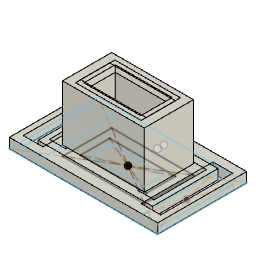
DrVape_DrStick v1 (Autodesk Fusion 360 design; units mm, degrees)
Autodesk Fusion 360 part; units mm, degrees
sketch "スケッチ1" plane through (0, 0, 0) normal (0, 0, 1) x (1, 0, 0)
  line L0 (7.7, 3.8) -> (-7.7, 3.8)
  line L1 (-7.7, 3.8) -> (-7.7, -3.8)
  line L2 (-7.7, -3.8) -> (7.7, -3.8)
  line L3 (7.7, -3.8) -> (7.7, 3.8)
  line L4 (7.7, 3.8) -> (-7.7, -3.8) construction
  line L5 (-7.7, 3.8) -> (7.7, -3.8) construction
  line L6 (10, -6) -> (-10, -6)
  line L7 (-10, -6) -> (-10, 6)
  line L8 (-10, 6) -> (10, 6)
  line L9 (10, 6) -> (10, -6)
  line L10 (10, -6) -> (-10, 6) construction
  line L11 (-10, -6) -> (10, 6) construction
  line L12 (17.5, -10) -> (-17.5, -10)
  line L13 (-17.5, -10) -> (-17.5, 10)
  line L14 (-17.5, 10) -> (17.5, 10)
  line L15 (17.5, 10) -> (17.5, -10)
  line L16 (17.5, -10) -> (-17.5, 10) construction
  line L17 (-17.5, -10) -> (17.5, 10) construction
  dimension "d1" = 15.4
  dimension "d2" = 7.6
  dimension "d3" = 20
  dimension "d4" = 12
  dimension "d5" = 35
  dimension "d6" = 20
  constraint horizontal L0
  constraint perpendicular L0 L1
  constraint parallel L0 L2
  constraint parallel L1 L3
  constraint coincident L4 origin
  constraint coincident L5 origin
  constraint horizontal L6
  constraint perpendicular L6 L7
  constraint parallel L6 L8
  constraint parallel L7 L9
  constraint coincident L10 origin
  constraint coincident L11 origin
  constraint horizontal L12
  constraint perpendicular L12 L13
  constraint parallel L12 L14
  constraint parallel L13 L15
  constraint coincident L16 origin
  constraint coincident L17 origin
  measures "d1" distance of L1.end L2.end
  measures "d2" distance of L0.end L1.end
  measures "d3" distance of L7.end L8.end
  measures "d4" distance of L6.end L7.end
  measures "d5" distance of L13.end L14.end
  measures "d6" distance of L12.end L13.end
extrude "押し出し1" add sketch "スケッチ1" along normal blind 20 contours L6 L7 L8 L9 makes body 1
extrude "押し出し2" add sketch "スケッチ1" along normal blind 3 contours L0 L1 L2 L3 | L6 L7 L8 L9 | L12 L13 L14 L15 bodies 1
chamfer "面取り1" distance 1 angle 45 4 edges at (0, 3.8, 20) (-7.7, 0, 20) (0, -3.8, 20) (7.7, 0, 20) on bodies 1
sketch "スケッチ2" plane through (0, 0, 3) normal (0, 0, 1) x (-1, 0, 0)
  line L0 (-17.5, -10) -> (17.5, -10)
  line L1 (17.5, -10) -> (17.5, 10)
  line L2 (17.5, 10) -> (-17.5, 10)
  line L3 (-17.5, 10) -> (-17.5, -10)
  line L4 (-10, -6) -> (-10, 6)
  line L5 (-10, 6) -> (10, 6)
  line L6 (10, 6) -> (10, -6)
  line L7 (10, -6) -> (-10, -6)
  line L8 (-11, -8) -> (-16, -8)
  line L9 (-16, -8) -> (-16, 8)
  line L10 (-16, 8) -> (-11, 8)
  line L11 (-11, 8) -> (-11, -8)
  line L12 (0, -7) -> (0, -1)
  line L13 (11, 8) -> (11, -8)
  line L14 (11, -8) -> (16, -8)
  line L15 (16, -8) -> (16, 8)
  line L16 (16, 8) -> (11, 8)
  line L17 (-6, 2) -> (6, 2)
  line L18 (6, 2) -> (6, -2)
  line L19 (6, -2) -> (-6, -2)
  line L20 (-6, -2) -> (-6, 2)
  line L21 (-6, 2) -> (6, -2) construction
  line L22 (6, 2) -> (-6, -2) construction
  constraint horizontal L8
  constraint vertical L9
  constraint horizontal L10
  constraint vertical L11
  constraint perpendicular L7 L12
  constraint symmetric L8.start L12 L13.end
  constraint symmetric L8.end L12 L14.end
  constraint symmetric L9.end L12 L15.end
  constraint symmetric L10.end L12 L13.start
  constraint horizontal L17
  constraint perpendicular L17 L18
  constraint parallel L17 L19
  constraint parallel L18 L20
  constraint coincident L21 origin
  constraint coincident L22 origin
extrude "押し出し3" cut sketch "スケッチ2" against normal blind 8 contours L8 L9 L10 L11 | L13 L14 L15 L16 | L17 L18 L19 L20 bodies 1
sketch "スケッチ3" plane through (0, 0, 0) normal (0, 0, 1) x (1, 0, 0)
  line L0 (10.05, -4.45) -> (-10.05, -4.45)
  line L1 (-10.05, -4.45) -> (-10.05, 4.45)
  line L2 (-10.05, 4.45) -> (10.05, 4.45)
  line L3 (10.05, 4.45) -> (10.05, -4.45)
  line L4 (10.05, -4.45) -> (-10.05, 4.45) construction
  line L5 (-10.05, -4.45) -> (10.05, 4.45) construction
  line L6 (12.5, 7.5) -> (-12.5, 7.5)
  line L7 (-12.5, 7.5) -> (-12.5, -7.5)
  line L8 (-12.5, -7.5) -> (12.5, -7.5)
  line L9 (12.5, -7.5) -> (12.5, 7.5)
  line L10 (12.5, 7.5) -> (-12.5, -7.5) construction
  line L11 (-12.5, 7.5) -> (12.5, -7.5) construction
  line L12 (8, -3) -> (-8, -3)
  line L13 (-8, -3) -> (-8, 3)
  line L14 (-8, 3) -> (8, 3)
  line L15 (8, 3) -> (8, -3)
  line L16 (8, -3) -> (-8, 3) construction
  line L17 (-8, -3) -> (8, 3) construction
  line L18 (22.6666, -13.6) -> (-22.6666, -13.6)
  line L19 (-22.6666, -13.6) -> (-22.6666, 13.6)
  line L20 (-22.6666, 13.6) -> (22.6666, 13.6)
  line L21 (22.6666, 13.6) -> (22.6666, -13.6)
  line L22 (22.6666, -13.6) -> (-22.6666, 13.6) construction
  line L23 (-22.6666, -13.6) -> (22.6666, 13.6) construction
  line L24 (21, -11) -> (15, -11)
  line L25 (15, -11) -> (15, 11)
  line L26 (15, 11) -> (21, 11)
  line L27 (21, 11) -> (21, -11)
  line L28 (21, -11) -> (15, 11) construction
  line L29 (15, -11) -> (21, 11) construction
  line L30 (0, 11) -> (0, 9)
  line L31 (-15, -11) -> (-15, 11)
  line L32 (-15, 11) -> (-21, 11)
  line L33 (-21, 11) -> (-21, -11)
  line L34 (-21, -11) -> (-15, -11)
  point P0 (18, 0)
  dimension "d14" = 20.1
  dimension "d15" = 8.9
  dimension "d16" = 25
  dimension "d17" = 15
  constraint horizontal L0
  constraint perpendicular L0 L1
  constraint parallel L0 L2
  constraint parallel L1 L3
  constraint coincident L4 origin
  constraint coincident L5 origin
  constraint horizontal L6
  constraint perpendicular L6 L7
  constraint parallel L6 L8
  constraint parallel L7 L9
  constraint coincident L10 origin
  constraint coincident L11 origin
  constraint horizontal L12
  constraint perpendicular L12 L13
  constraint parallel L12 L14
  constraint parallel L13 L15
  constraint coincident L16 origin
  constraint coincident L17 origin
  constraint horizontal L18
  constraint perpendicular L18 L19
  constraint parallel L18 L20
  constraint parallel L19 L21
  constraint coincident L22 origin
  constraint coincident L23 origin
  constraint horizontal L24
  constraint perpendicular L24 L25
  constraint parallel L24 L26
  constraint parallel L25 L27
  constraint coincident L28 P0
  constraint coincident L29 P0
  constraint perpendicular L20 L30
  constraint symmetric L24.start L30 L33.end
  constraint symmetric L24.end L30 L31.start
  constraint symmetric L25.end L30 L31.end
  constraint symmetric L26.end L30 L32.end
  measures "d14" distance of L1.end L2.end
  measures "d15" distance of L0.end L1.end
  measures "d16" distance of L7.end L8.end
  measures "d17" distance of L6.end L7.end
extrude "押し出し4" add sketch "スケッチ3" along normal blind 20 separate body contours L6 L7 L8 L9 makes body 2
extrude "押し出し5" add sketch "スケッチ3" along normal blind 3 bodies 2
named bodies: "Dr.Stick", "DR,Vape"
